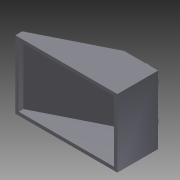
# Autodesk Inventor part: LEGO Brick 3298
Saved by Autodesk Inventor 2011 SP1 (Build 150282100, 282)
## iProperties
Company: Allseas Engineering BV
Created: 2011-09-27
Part Number: LEGO Brick 3298
Cost Center: 0 kg
Material: Steel
Document SubType Name: Modeling
Designer: BvH
Authority: 0 mm^3
Stock Number: =<Filenr>_<Document number>
Density: 7.85 g/cm^3
Act. Code: DW000
SaveDate: 2011-07-28
SaveTime: 18:32
FileName: Standard
TotalMass: 0 kg
TotalVolume: 0 mm^3
Subject: =<Title><TITLE 1_2> <TITLE 2_2>
Author: BvH
Autodesk Inventor part; units mm, degrees
ref_plane "YZ Plane" through (0, 0, 0) normal (1, 0, 0) x (0, 1, 0)
ref_plane "XZ Plane" through (0, 0, 0) normal (0, 1, 0) x (-1, 0, 0)
ref_plane "XY Plane" through (0, 0, 0) normal (0, 0, 1) x (1, 0, 0)
sketch "Sketch1" plane through (0, 0, 0) normal (0, 0, 1) x (1, 0, 0)
  line L0 (12, 0) -> (-12, 0)
  line L1 (-12, 0) -> (-12, 1.6)
  line L2 (-12, 1.6) -> (4, 9.6)
  line L3 (4, 9.6) -> (12, 9.6)
  line L4 (12, 9.6) -> (12, 0)
  point P0 (0, 0)
  point P1 (0, 0)
  dimension "d0" = 9.6
  dimension "d1" = 24
  dimension "d2" = 16
  dimension "d3" = 1.6
  constraints: 10 end point, 2 horizontal, 2 vertical, 1 coincident, 1 midpoint
  measures "d0" distance between parallel lines of L0 L3
  measures "d1" distance between parallel lines of L4 L1
  measures "d2" distance from line of L2.end L1
  measures "d3" distance of L0.end L1.end
extrude "Extrusion1" add sketch "Sketch1" along normal mid plane 16
shell "Shell1" thickness 0.8 removed faces 1 at (-4, 0, 2.6667)
sketch "Sketch2" plane through (4, 9.6, 8) normal (0, 1, 0) x (1, 0, 0)
  line L0 (4, 12) -> (4, 4) construction
  line L1 (-20.8, 8) -> (12.8, 8) construction
  line L2 (8, 0) -> (8, 16) construction
  circle A0 centre (4, 12) radius 2.5
  circle A1 centre (4, 4) radius 2.5
  point P0 (4, 8)
  dimension "d6" = 4
  dimension "d7" = 8
  dimension "d8" = 5
  constraints: 2 centre point, 2 coincident, 2 end point, 1 equal radius, 1 midpoint, 1 point on line, 1 vertical
  measures "d6" distance between parallel lines of L2 L0
  measures "d7" distance of L0.start L0.end
  measures "d8" diameter of A0
extrude "Extrusion2" add sketch "Sketch2" along normal blind 1.6
body "Solid1"
